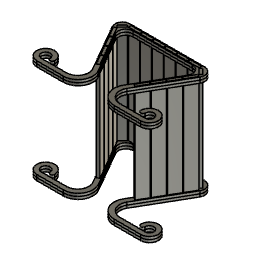
kollur (Autodesk Fusion 360 design; units mm, degrees)
Autodesk Fusion 360 part; units mm, degrees
sketch "Sketch1" plane through (0, 0, 0) normal (0, 0, 1) x (1, 0, 0)
  line L0 (113.7474, 37.6527) -> (283.8436, 37.6527)
  line L1 (348.7955, 150.1527) -> (168.3735, 462.6527)
  line L2 (211.6748, 537.6527) -> (463.7474, 537.6527)
  line L3 (379.1064, 157.6527) -> (220.335, 432.6527)
  line L4 (233.163, 537.6527) -> (233.163, 487.6527)
  line L5 (263.6363, 507.6527) -> (463.7474, 507.6527)
  line L6 (113.7474, 7.6527) -> (292.5038, 7.6527)
  arc A0 (263.6363, 507.6527) -> (220.335, 432.6527) centre (263.6363, 457.6527) ccw
  arc A1 (211.6748, 537.6527) -> (168.3735, 462.6527) centre (211.6748, 487.6527) ccw
  arc A2 (283.8436, 37.6527) -> (348.7955, 150.1527) centre (283.8436, 112.6527) ccw
  arc A3 (292.5038, 7.6527) -> (379.1064, 157.6527) centre (292.5038, 107.6527) ccw
  line L7 (113.7474, 7.6527) -> (463.7474, 7.6527)
  line L8 (463.7474, 7.6527) -> (463.7474, 700)
  line L9 (548.3884, 157.6527) -> (707.1597, 432.6527)
  line L10 (694.3317, 537.6527) -> (694.3317, 487.6527)
  line L11 (813.7474, 37.6527) -> (643.6512, 37.6527)
  line L12 (813.7474, 37.6527) -> (813.7474, 7.6527)
  line L13 (578.6993, 150.1527) -> (759.1212, 462.6527)
  arc A4 (548.3884, 157.6527) -> (634.9909, 7.6527) centre (634.9909, 107.6527) ccw
  arc A5 (759.1212, 462.6527) -> (715.82, 537.6527) centre (715.82, 487.6527) ccw
  arc A6 (707.1597, 432.6527) -> (663.8584, 507.6527) centre (663.8584, 457.6527) ccw
  line L14 (813.7474, 7.6527) -> (634.9909, 7.6527)
  arc A7 (578.6993, 150.1527) -> (643.6512, 37.6527) centre (643.6512, 112.6527) ccw
  line L15 (663.8584, 507.6527) -> (463.7474, 507.6527)
  line L16 (715.82, 537.6527) -> (463.7474, 537.6527)
  line L17 (226.2474, 531.6527) -> (463.7474, 531.6527)
  line L18 (226.2474, 513.6527) -> (463.7474, 513.6527)
  line L19 (226.2474, 531.6527) -> (226.2474, 513.6527)
  line L20 (701.2474, 531.6527) -> (463.7474, 531.6527)
  line L21 (701.2474, 531.6527) -> (701.2474, 513.6527)
  line L22 (701.2474, 513.6527) -> (463.7474, 513.6527)
  line L23 (301.2474, 531.6527) -> (301.2474, 513.6527)
  line L24 (381.2474, 531.6527) -> (381.2474, 513.6527)
  line L25 (306.2474, 531.6527) -> (306.2474, 513.6527)
  line L26 (386.2474, 531.6527) -> (386.2474, 513.6527)
  line L27 (461.2474, 531.6527) -> (461.2474, 513.6527)
  line L28 (626.2474, 531.6527) -> (626.2474, 513.6527)
  line L29 (621.2474, 531.6527) -> (621.2474, 513.6527)
  line L30 (546.2474, 531.6527) -> (546.2474, 513.6527)
  line L31 (541.2474, 531.6527) -> (541.2474, 513.6527)
  line L32 (466.2474, 531.6527) -> (466.2474, 513.6527)
  line L33 (113.7474, 37.6527) -> (113.7474, 67.6527)
  arc A8 (143.7474, 67.6527) -> (113.7474, 37.6527) centre (113.7474, 67.6527) ccw
  arc A9 (173.7474, 67.6527) -> (113.7474, 7.6527) centre (113.7474, 67.6527) ccw
  arc A10 (143.7474, 67.6527) -> (173.7474, 67.6527) centre (158.7474, 67.6527) ccw
  arc A11 (813.7474, 7.6527) -> (753.7474, 67.6527) centre (813.7474, 67.6527) ccw
  arc A12 (813.7474, 37.6527) -> (783.7474, 67.6527) centre (813.7474, 67.6527) ccw
  arc A13 (753.7474, 67.6527) -> (783.7474, 67.6527) centre (768.7474, 67.6527) ccw
  point P0 (413.7474, 37.6527)
  point P1 (125.0722, 537.6527)
  point P2 (607.0486, 65)
  point P3 (802.4225, 537.6527)
  point P4 (513.7474, 37.6527)
  point P5 (927.4947, 0)
  dimension "d1" = 300
  dimension "d2" = 500
  dimension "d3" = 60
  dimension "d4" = 30
  dimension "d8" = 50
  dimension "d9" = 50
  dimension "d10" = 50
  dimension "d13" = 75
  dimension "d14" = 60
  dimension "d15" = 100
  dimension "d18" = 30
  dimension "d19" = 30
  dimension "d21" = 350
  dimension "d24" = 6
  dimension "d25" = 6
  dimension "d26" = 237.5
  dimension "d31" = 75
  dimension "d32" = 5
  dimension "d33" = 75
  dimension "d34" = 5
  dimension "d35" = 75
  dimension "d36" = 30
  dimension "d37" = 30
  constraint horizontal L0
  constraint parallel L1 L3
  constraint coincident L2 L4.start
  constraint perpendicular L2 L4
  constraint horizontal L5
  constraint tangent L3 A0
  constraint tangent L5 A0
  constraint coincident P1 L2
  constraint coincident P1 L1
  constraint tangent L2 A1
  constraint tangent L1 A1
  constraint coincident P0 L1
  constraint coincident P0 L0
  constraint tangent L1 A2
  constraint tangent L0 A2
  constraint tangent L3 A3
  constraint tangent L6 A3
  constraint perpendicular L2 L8
  constraint coincident L8 L2.end
  constraint coincident L8 L5.end
  constraint symmetric origin L8 P5
  constraint symmetric L0.start L8 L11.start
  constraint symmetric P0 L8 P4
  constraint symmetric P1 L8 P3
  constraint symmetric L6.start L8 L12.end
  constraint symmetric L4.start L8 L10.start
  constraint symmetric L4.end L8 L10.end
  constraint symmetric L3.end L8 L9.end
  constraint symmetric L5.start L8 A6.end
  constraint symmetric A0 L8 A6
  constraint symmetric L2.start L8 A5.end
  constraint symmetric L1.end L8 L13.end
  constraint symmetric A1 L8 A5
  constraint symmetric L1.start L8 L13.start
  constraint symmetric L0.end L8 L11.end
  constraint symmetric A2 L8 A7
  constraint symmetric L3.start L8 L9.start
  constraint symmetric L6.end L8 A4.end
  constraint symmetric A3 L8 A4
  constraint symmetric L8 L2.end L16.end
  constraint symmetric L8 L5.end L15.end
  constraint coincident L8 L17.end
  constraint perpendicular L8 L17
  constraint coincident L8 L18.end
  constraint perpendicular L8 L18
  constraint perpendicular L18 L19
  constraint symmetric L8 L17.start L20.start
  constraint symmetric L8 L17.end L20.end
  constraint symmetric L8 L18.start L21.end
  constraint symmetric L8 L18.end L22.end
  constraint coincident L17 L23.start
  constraint coincident L18 L23.end
  constraint perpendicular L18 L23
  constraint coincident L17 L24.start
  constraint coincident L18 L24.end
  constraint perpendicular L18 L24
  constraint coincident L17 L25.start
  constraint coincident L18 L25.end
  constraint perpendicular L18 L25
  constraint coincident L17 L26.start
  constraint coincident L18 L26.end
  constraint perpendicular L18 L26
  constraint coincident L17 L27.start
  constraint coincident L18 L27.end
  constraint perpendicular L18 L27
  constraint symmetric L8 L23.start L28.start
  constraint symmetric L8 L23.end L28.end
  constraint symmetric L8 L24.start L30.start
  constraint symmetric L8 L24.end L30.end
  constraint symmetric L8 L25.start L29.start
  constraint symmetric L8 L25.end L29.end
  constraint symmetric L8 L26.start L31.start
  constraint symmetric L8 L26.end L31.end
  constraint symmetric L8 L27.start L32.start
  constraint symmetric L8 L27.end L32.end
  constraint perpendicular L0 L33
  constraint coincident L33.end A8.centre
  constraint concentric A8 A9
  constraint symmetric L8 A9.start A11.end
  constraint symmetric L8 A8.start A12.end
  constraint symmetric L8 A8 A12
  constraint symmetric L8 A9 A11
  constraint symmetric L8 A10 A13
  measures "d1" distance of L0.start P0
  measures "d2" vertical distance of L0.start P1
  measures "d3" angle of L0 L1
  measures "d4" distance of L0.start L6.start
  measures "d8" distance of L4.start L4.end
  measures "d9" radius of A0
  measures "d10" radius of A1
  measures "d13" radius of A2
  measures "d14" angle of L3 L6
  measures "d15" radius of A3
  measures "d18" distance of L2 L5
  measures "d19" distance of L1 L3
  measures "d21" distance of L6.start L7.end
  measures "d24" distance of L2 L17
  measures "d25" distance of L5 L18
  measures "d26" distance of L8 L19
  measures "d31" distance of L19 L23
  measures "d32" distance of L23 L25
  measures "d33" distance of L24 L25
  measures "d34" distance of L24 L26
  measures "d35" distance of L26 L27
  measures "d36" distance of L0.start L33.end
  measures "d37" diameter of A10
extrude "Extrude1" add sketch "Sketch1" along normal blind 18 contours L0 L1 L2 L3 L4 L6 A0 A1 A2 A3 L7 L17 L18 L19 A8 A9 A10 | L2 L4 L8 L17 | L8 L10 L16 L20 | L4 L5 A0 L8 L18 | L8 L10 A6 L15 L22 | L8 L20 L22 L32 | L8 L17 L18 L27 | L9 L10 L11 L12 L13 A4 A5 A6 L14 A7 L16 L20 L21 L22 | L17 L18 L23 L25 | L17 L18 L24 L26 | L20 L22 L30 L31 | L20 L22 L28 L29 | L12 A11 A12 A13 makes body 1
copy_body "CopyPasteBodies1" bodies 1 makes body 2
move_body "Move1" bodies 2 to x (1, 0, 0) y (0, 1, 0) z (0, 0, 1) at (0, 0, 18)
copy_body "CopyPasteBodies2" bodies 2 1 makes body 3 makes body 4
move_body "Move2" bodies 3 4 to x (1, 0, 0) y (0, 1, 0) z (0, 0, 1) at (0, 0, 636)
move_body "Move3" bodies 1 2 to x (1, 0, 0) y (0, 1, 0) z (0, 0, 1) at (0, 0, -28)
move_body "Align1" bodies 3 to x (1, 0, 0) y (0, 1, 0) z (0, 0, 1) at (0, 0, 0)
move_body "Align2" bodies 1 to x (1, 0, 0) y (0, 1, 0) z (0, 0, 1) at (0, 0, 0)
sketch "Sketch2" plane through (0, 0, 0) normal (0, 1, 0) x (1, 0, 0)
  line L0 (-100, -350) -> (-100, 250)
  line L1 (-100, 250) -> (-175, 250)
  line L2 (-175, 250) -> (-175, -350)
  line L3 (-175, -350) -> (-100, -350)
  dimension "d38" = 600
  dimension "d39" = 75
  constraint vertical L0
  constraint perpendicular L0 L1
  constraint perpendicular L1 L2
  constraint perpendicular L0 L3
  measures "d38" distance of L0.start L0.end
  measures "d39" distance of L0.end L1.end
sketch "Sketch3" plane through (0, 0, -28) normal (0, 0, -1) x (1, 0, 0)
  line L0 (701.2474, -531.6527) -> (626.2474, -531.6527)
  line L1 (626.2474, -531.6527) -> (626.2474, -513.6527)
  line L2 (626.2474, -513.6527) -> (701.2474, -513.6527)
  line L3 (701.2474, -513.6527) -> (701.2474, -531.6527)
  line L4 (226.2474, -531.6527) -> (226.2474, -513.6527)
  line L5 (226.2474, -513.6527) -> (301.2474, -513.6527)
  line L6 (301.2474, -513.6527) -> (301.2474, -531.6527)
  line L7 (301.2474, -531.6527) -> (226.2474, -531.6527)
  line L8 (541.2474, -531.6527) -> (466.2474, -531.6527)
  line L9 (466.2474, -531.6527) -> (466.2474, -513.6527)
  line L10 (466.2474, -513.6527) -> (541.2474, -513.6527)
  line L11 (541.2474, -513.6527) -> (541.2474, -531.6527)
  line L12 (386.2474, -531.6527) -> (386.2474, -513.6527)
  line L13 (386.2474, -513.6527) -> (461.2474, -513.6527)
  line L14 (461.2474, -513.6527) -> (461.2474, -531.6527)
  line L15 (461.2474, -531.6527) -> (386.2474, -531.6527)
  line L16 (381.2474, -531.6527) -> (306.2474, -531.6527)
  line L17 (306.2474, -531.6527) -> (306.2474, -513.6527)
  line L18 (306.2474, -513.6527) -> (381.2474, -513.6527)
  line L19 (381.2474, -513.6527) -> (381.2474, -531.6527)
  line L20 (621.2474, -531.6527) -> (546.2474, -531.6527)
  line L21 (546.2474, -531.6527) -> (546.2474, -513.6527)
  line L22 (546.2474, -513.6527) -> (621.2474, -513.6527)
  line L23 (621.2474, -513.6527) -> (621.2474, -531.6527)
  arc A0 (753.7474, -67.6527) -> (813.7474, -7.6527) centre (813.7474, -67.6527) ccw
  line L24 (813.7474, -7.6527) -> (634.9909, -7.6527)
  arc A1 (634.9909, -7.6527) -> (548.3884, -157.6527) centre (634.9909, -107.6527) ccw
  line L25 (548.3884, -157.6527) -> (707.1597, -432.6527)
  arc A2 (663.8584, -507.6527) -> (707.1597, -432.6527) centre (663.8584, -457.6527) ccw
  line L26 (663.8584, -507.6527) -> (263.6363, -507.6527)
  arc A3 (220.335, -432.6527) -> (263.6363, -507.6527) centre (263.6363, -457.6527) ccw
  line L27 (220.335, -432.6527) -> (379.1064, -157.6527)
  arc A4 (379.1064, -157.6527) -> (292.5038, -7.6527) centre (292.5038, -107.6527) ccw
  line L28 (292.5038, -7.6527) -> (113.7474, -7.6527)
  arc A5 (113.7474, -7.6527) -> (173.7474, -67.6527) centre (113.7474, -67.6527) ccw
  arc A6 (173.7474, -67.6527) -> (143.7474, -67.6527) centre (158.7474, -67.6527) ccw
  arc A7 (113.7474, -37.6527) -> (143.7474, -67.6527) centre (113.7474, -67.6527) ccw
  line L29 (113.7474, -37.6527) -> (283.8436, -37.6527)
  arc A8 (348.7955, -150.1527) -> (283.8436, -37.6527) centre (283.8436, -112.6527) ccw
  line L30 (348.7955, -150.1527) -> (168.3735, -462.6527)
  arc A9 (168.3735, -462.6527) -> (211.6748, -537.6527) centre (211.6748, -487.6527) ccw
  line L31 (211.6748, -537.6527) -> (715.82, -537.6527)
  arc A10 (715.82, -537.6527) -> (759.1212, -462.6527) centre (715.82, -487.6527) ccw
  line L32 (759.1212, -462.6527) -> (578.6993, -150.1527)
  arc A11 (643.6512, -37.6527) -> (578.6993, -150.1527) centre (643.6512, -112.6527) ccw
  line L33 (643.6512, -37.6527) -> (813.7474, -37.6527)
  arc A12 (783.7474, -67.6527) -> (813.7474, -37.6527) centre (813.7474, -67.6527) ccw
  arc A13 (783.7474, -67.6527) -> (753.7474, -67.6527) centre (768.7474, -67.6527) ccw
  line L34 (701.2474, -531.6527) -> (626.2474, -531.6527)
  line L35 (626.2474, -531.6527) -> (626.2474, -513.6527)
  line L36 (626.2474, -513.6527) -> (701.2474, -513.6527)
  line L37 (701.2474, -513.6527) -> (701.2474, -531.6527)
  line L38 (621.2474, -531.6527) -> (546.2474, -531.6527)
  line L39 (546.2474, -531.6527) -> (546.2474, -513.6527)
  line L40 (546.2474, -513.6527) -> (621.2474, -513.6527)
  line L41 (621.2474, -513.6527) -> (621.2474, -531.6527)
  line L42 (541.2474, -531.6527) -> (466.2474, -531.6527)
  line L43 (466.2474, -531.6527) -> (466.2474, -513.6527)
  line L44 (466.2474, -513.6527) -> (541.2474, -513.6527)
  line L45 (541.2474, -513.6527) -> (541.2474, -531.6527)
  line L46 (461.2474, -531.6527) -> (386.2474, -531.6527)
  line L47 (386.2474, -531.6527) -> (386.2474, -513.6527)
  line L48 (386.2474, -513.6527) -> (461.2474, -513.6527)
  line L49 (461.2474, -513.6527) -> (461.2474, -531.6527)
  line L50 (381.2474, -531.6527) -> (306.2474, -531.6527)
  line L51 (306.2474, -531.6527) -> (306.2474, -513.6527)
  line L52 (306.2474, -513.6527) -> (381.2474, -513.6527)
  line L53 (381.2474, -513.6527) -> (381.2474, -531.6527)
  line L54 (301.2474, -531.6527) -> (226.2474, -531.6527)
  line L55 (226.2474, -531.6527) -> (226.2474, -513.6527)
  line L56 (226.2474, -513.6527) -> (301.2474, -513.6527)
  line L57 (301.2474, -513.6527) -> (301.2474, -531.6527)
  line L58 (701.2474, -513.6527) -> (757.8159, -457.0842)
  line L59 (701.2474, -513.6527) -> (781.2474, -513.6527) construction
  line L60 (701.2474, -513.6527) -> (704.7829, -510.1172)
  line L61 (704.7829, -510.1172) -> (717.5108, -522.8451)
  line L62 (717.5108, -522.8451) -> (752.8662, -487.4898)
  line L63 (752.8662, -487.4898) -> (740.1382, -474.7618)
  line L64 (463.7474, -537.6527) -> (463.7474, -507.6527)
  line L65 (209.9839, -522.8451) -> (174.6286, -487.4898)
  line L66 (222.7118, -510.1172) -> (209.9839, -522.8451)
  line L67 (226.2474, -513.6527) -> (169.6788, -457.0842)
  line L68 (174.6286, -487.4898) -> (187.3565, -474.7618)
  line L69 (751.9227, -462.1846) -> (714.4227, -397.2327)
  line L70 (714.4227, -397.2327) -> (698.8343, -406.2327)
  line L71 (698.8343, -406.2327) -> (736.3343, -471.1846)
  line L72 (736.3343, -471.1846) -> (751.9227, -462.1846)
  line L73 (697.4074, -404.1697) -> (713.3806, -394.9476)
  line L74 (658.8343, -336.9506) -> (674.4227, -327.9506)
  line L75 (674.4227, -327.9506) -> (711.9227, -392.9025)
  line L76 (696.3343, -401.9025) -> (658.8343, -336.9506)
  line L77 (711.9227, -392.9025) -> (696.3343, -401.9025)
  line L78 (661.4683, -332.5431) -> (672.2839, -326.2988)
  line L79 (578.8343, -198.3866) -> (594.4227, -189.3866)
  line L80 (594.4227, -189.3866) -> (631.9227, -254.3385)
  line L81 (616.3343, -263.3385) -> (578.8343, -198.3866)
  line L82 (631.9227, -254.3385) -> (616.3343, -263.3385)
  line L83 (634.4227, -258.6686) -> (618.8343, -267.6686)
  line L84 (671.9227, -323.6205) -> (634.4227, -258.6686)
  line L85 (618.8343, -267.6686) -> (656.3343, -332.6205)
  line L86 (656.3343, -332.6205) -> (671.9227, -323.6205)
  line L87 (228.6605, -406.2327) -> (191.1605, -471.1846)
  line L88 (191.1605, -471.1846) -> (175.572, -462.1846)
  line L89 (175.572, -462.1846) -> (213.072, -397.2327)
  line L90 (213.072, -397.2327) -> (228.6605, -406.2327)
  line L91 (215.572, -392.9025) -> (231.1605, -401.9025)
  line L92 (253.072, -327.9506) -> (215.572, -392.9025)
  line L93 (231.1605, -401.9025) -> (268.6605, -336.9506)
  line L94 (268.6605, -336.9506) -> (253.072, -327.9506)
  line L95 (271.1605, -332.6205) -> (255.572, -323.6205)
  line L96 (255.572, -323.6205) -> (293.072, -258.6686)
  line L97 (308.6605, -267.6686) -> (271.1605, -332.6205)
  line L98 (293.072, -258.6686) -> (308.6605, -267.6686)
  line L99 (333.072, -189.3866) -> (295.572, -254.3385)
  line L100 (295.572, -254.3385) -> (311.1605, -263.3385)
  line L101 (311.1605, -263.3385) -> (348.6605, -198.3866)
  line L102 (348.6605, -198.3866) -> (333.072, -189.3866)
  dimension "d44" = 80
  dimension "d45" = 45
  dimension "d46" = 5
  dimension "d47" = 18
  dimension "d48" = 50
  dimension "d49" = 75
  dimension "d50" = 18
  dimension "d51" = 75
  dimension "d52" = 6
  dimension "d53" = 5
  dimension "d54" = 2.5
  dimension "d55" = 2.5
  constraint horizontal L34
  constraint vertical L35
  constraint horizontal L36
  constraint vertical L37
  constraint coincident L1.end L2.start
  constraint coincident L0.start L3.end
  constraint horizontal L38
  constraint vertical L39
  constraint horizontal L40
  constraint vertical L41
  constraint coincident L21.end L22.start
  constraint coincident L20.start L23.end
  constraint horizontal L42
  constraint vertical L43
  constraint horizontal L44
  constraint vertical L45
  constraint coincident L9.end L10.start
  constraint coincident L8.start L11.end
  constraint horizontal L46
  constraint vertical L47
  constraint horizontal L48
  constraint vertical L49
  constraint coincident L12.end L13.start
  constraint coincident L14.end L15.start
  constraint horizontal L50
  constraint vertical L51
  constraint horizontal L52
  constraint vertical L53
  constraint coincident L17.end L18.start
  constraint coincident L16.start L19.end
  constraint horizontal L54
  constraint vertical L55
  constraint horizontal L56
  constraint vertical L57
  constraint coincident L4.end L5.start
  constraint coincident L6.end L7.start
  constraint horizontal L59
  constraint parallel L58 L60
  constraint perpendicular L58 L61
  constraint perpendicular L61 L62
  constraint coincident L58 L63.end
  constraint perpendicular L58 L63
  constraint midpoint L31 L64.start
  constraint midpoint L26 L64.end
  constraint symmetric L2.end L64 L4.end
  constraint symmetric L58.end L64 L67.end
  constraint symmetric L60.end L64 L66.start
  constraint symmetric L61.end L64 L65.start
  constraint symmetric L62.end L64 L65.end
  constraint symmetric L63.end L64 L68.end
  constraint parallel L32 L69
  constraint perpendicular L25 L70
  constraint perpendicular L70 L71
  constraint perpendicular L25 L73
  constraint symmetric L69.start L73 L74.end
  constraint symmetric L69.end L73 L75.end
  constraint symmetric L70.end L73 L76.start
  constraint symmetric L71.end L73 L74.start
  constraint perpendicular L32 L78
  constraint symmetric L69.start L78 L79.end
  constraint symmetric L69.end L78 L80.end
  constraint symmetric L70.end L78 L81.start
  constraint symmetric L71.end L78 L79.start
  constraint symmetric L74.start L78 L85.end
  constraint symmetric L74.end L78 L84.start
  constraint symmetric L75.end L78 L83.start
  constraint symmetric L76.start L78 L83.end
  constraint symmetric L64 L69.start L88.end
  constraint symmetric L64 L69.end L89.end
  constraint symmetric L64 L70.end L87.start
  constraint symmetric L64 L71.end L87.end
  constraint symmetric L64 L74.start L93.end
  constraint symmetric L64 L74.end L92.start
  constraint symmetric L64 L75.end L91.start
  constraint symmetric L64 L76.start L91.end
  constraint symmetric L64 L79.start L101.end
  constraint symmetric L64 L79.end L99.start
  constraint symmetric L64 L80.end L99.end
  constraint symmetric L64 L81.start L100.end
  constraint symmetric L64 L83.start L96.end
  constraint symmetric L64 L83.end L97.start
  constraint symmetric L64 L84.start L95.end
  constraint symmetric L64 L85.end L95.start
  measures "d44" distance of L2.end L58.end
  measures "d45" angle of L58 L59
  measures "d46" distance of L2.end L60.end
  measures "d47" distance of L60.end L61.end
  measures "d48" distance of L61.end L62.end
  measures "d49" distance of L69.start L69.end
  measures "d50" distance of L69.end L70.end
  measures "d51" distance of L70.end L71.end
  measures "d52" distance of L32 L69
  measures "d53" distance of L63.end L72
  measures "d54" distance of L70 L73
  measures "d55" distance of L74 L78
extrude "Extrude3" cut sketch "Sketch3" against normal blind 700 contours L0 L1 L2 L3 L34 L35 L36 L37 | L4 L5 L6 L7 L54 L55 L56 L57 | L8 L9 L10 L11 L42 L43 L44 L45 | L12 L13 L14 L15 L46 L47 L48 L49 | L16 L17 L18 L19 L50 L51 L52 L53 | L20 L21 L22 L23 L38 L39 L40 L41 | L58 L61 L62 L63 | L65 L66 L67 L68 | L69 L70 L71 L72 | L74 L75 L76 L77 | L79 L80 L81 L82 | L83 L84 L85 L86 | L87 L88 L89 L90 | L91 L92 L93 L94 | L95 L96 L97 L98 | L99 L100 L101 L102 bodies 1 2 3 4
extrude "Extrude4" add sketch "Sketch3" against normal blind 700 separate body contours L0 L1 L2 L3 L34 L35 L36 L37 | L4 L5 L6 L7 L54 L55 L56 L57 | L8 L9 L10 L11 L42 L43 L44 L45 | L12 L13 L14 L15 L46 L47 L48 L49 | L16 L17 L18 L19 L50 L51 L52 L53 | L20 L21 L22 L23 L38 L39 L40 L41 | L58 L61 L62 L63 | L65 L66 L67 L68 | L69 L70 L71 L72 | L74 L75 L76 L77 | L79 L80 L81 L82 | L83 L84 L85 L86 | L87 L88 L89 L90 | L91 L92 L93 L94 | L95 L96 L97 L98 | L99 L100 L101 L102 makes body 5 at (240.572, 349.6013, 205.3333) makes body 6 at (356.2474, 531.6527, 205.3333) makes body 7 at (676.2474, 531.6527, 205.3333) makes body 8 at (683.8343, 380.2519, 205.3333) makes body 9 at (659.4227, 301.9699, 205.3333) makes body 10 at (516.2474, 531.6527, 205.3333) makes body 11 at (210.9267, 498.3321, 205.3333) makes body 12 at (268.072, 301.9699, 205.3333) makes body 13 at (188.072, 440.5339, 205.3333) makes body 14 at (411.2474, 513.6527, 205.3333) makes body 15 at (729.2959, 511.06, 438.6667) makes body 16 at (739.4227, 440.5339, 205.3333) makes body 17 at (606.9227, 211.0372, 205.3333) makes body 18 at (596.2474, 531.6527, 205.3333) makes body 19 at (251.2474, 513.6527, 205.3333) makes body 20 at (320.572, 211.0372, 438.6667)
